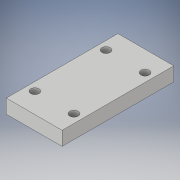
# Autodesk Inventor part: 20X20 carege
Saved by Autodesk Inventor 2019 (Build 230136000, 136)
## iProperties
Created: 2018-12-06
Part Number: 20X20 carege
Material: Generic
Document SubType Name: Modeling
Designer: User
Density: 1 g/cm^3
Appearance: Default
Author: User
Autodesk Inventor part; units mm, degrees
ref_plane "YZ Plane" through (0, 0, 0) normal (1, 0, 0) x (0, 1, 0)
ref_plane "XZ Plane" through (0, 0, 0) normal (0, 1, 0) x (-1, 0, 0)
ref_plane "XY Plane" through (0, 0, 0) normal (0, 0, 1) x (1, 0, 0)
sketch "Sketch1" plane through (0, 0, 0) normal (0, 1, 0) x (-1, 0, 0)
  line L0 (0, 0) -> (25.4, 0)
  line L1 (25.4, 0) -> (25.4, -50.8)
  line L2 (25.4, -50.8) -> (0, -50.8)
  line L3 (0, -50.8) -> (0, 0)
  dimension "d0" = 50.8
  dimension "d1" = 25.4
  constraints: 8 end point, 2 parallel, 1 horizontal, 1 perpendicular
  measures "d0" distance of L0.end L1.end
  measures "d1" distance of L1.end L2.end
extrude "Extrusion1" add sketch "Sketch1" along normal blind 6.35
sketch "Sketch2" plane through (0, 6.35, 0) normal (0, 1, 0) x (1, 0, 0)
  line L0 (-25.4, 0) -> (0, 0) projected
  line L1 (0, 0) -> (0, 50.8) projected
  line L2 (0, 50.8) -> (-25.4, 50.8) projected
  line L3 (-25.4, 50.8) -> (-25.4, 0) projected
  point P0 (-21.59, 9.2075)
  point P1 (-21.59, 41.5925)
  point P2 (-3.81, 9.2075)
  point P3 (-3.81, 41.5925)
  dimension "d4" = 32.385
  dimension "d5" = 50.8
  dimension "d6" = 9.2075
  dimension "d9" = 32.385
  dimension "d10" = 3.81
  dimension "d11" = 3.81
  dimension "d12" = 3.81
  dimension "d13" = 3.81
  dimension "d14" = 9.2075
  measures "d4" distance of point (-21.59, 41.593) point (-21.59, 9.207)
  measures "d5" distance of L2.end L0.start
  measures "d6" distance from line of point (-21.59, 9.207) L0
  measures "d9" distance of point (-3.81, 41.593) point (-3.81, 9.207)
  measures "d10" distance from line of L1 point (-3.81, 9.207)
  measures "d11" distance from line of L3 point (-21.59, 9.207)
  measures "d12" distance from line of L3 point (-21.59, 41.593)
  measures "d13" distance from line of L1 point (-3.81, 41.593)
  measures "d14" distance from line of L0 point (-3.81, 9.207)
hole "Hole1" at (-21.59, 6.35, -9.2075) at (-21.59, 6.35, -41.5925) at (-3.81, 6.35, -9.2075) at (-3.81, 6.35, -41.5925) direction (0, -1, 0) diameter 3.81 depth 25.4 tip angle 118
equation "\"d6\" = -0.5 * d4 + 0.5 * d5"
equation "\"d9\" = d4"
equation "\"d11\" = d10"
equation "\"d12\" = d10"
equation "\"d13\" = d10"
equation "\"d14\" = d6"
body "Solid1"
